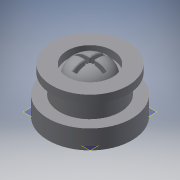
# Autodesk Inventor part: AX12_Idler
Saved by Autodesk Inventor 2017 (Build 210142000, 142)
## iProperties
Created: 2016-09-05
Part Number: AX12_Idler
Material: Generic
Document SubType Name: Modeling
Designer: Labtech
Density: 1 g/cm^3
Appearance: Default
Author: Labtech
Autodesk Inventor part; units mm, degrees
ref_plane "YZ Plane" through (0, 0, 0) normal (1, 0, 0) x (0, 1, 0)
ref_plane "XZ Plane" through (0, 0, 0) normal (0, 1, 0) x (-1, 0, 0)
sketch "Sketch1" plane through (0, 0, 0) normal (0, 0, 1) x (1, 0, 0)
  circle A0 centre (0, 0) radius 4 projected
  circle A1 centre (0, 0) radius 1.625 projected
  point P0 (0, 0)
ref_plane "Work Plane1" through (-11.5847, -11.5847, 5.5) normal (0, 0, 1) x (0.9999727, 0.0073902, 0)
extrude "Extrusion1" add sketch "Sketch1" along normal up to surface (5.5 mm away)
sketch "Sketch2" plane through (0, 0, 5.5) normal (0, 0, 1) x (1, 0, 0)
  circle A0 centre (0, 0) radius 3
  circle A1 centre (0, 0) radius 5
  dimension "d2" = 6
  dimension "d3" = 10
  constraints: 2 centre point, 2 coincident
  measures "d2" diameter of A0
  measures "d3" diameter of A1
extrude "Extrusion2" add sketch "Sketch2" along normal blind 1
ref_plane "Work Plane2" through (0, 0, 1) normal (0, 0, -1) x (-1, 0, 0)
sketch "Sketch3" plane through (0, 0, 1) normal (0, 0, -1) x (-1, 0, 0)
  circle A0 centre (0, 0) radius 4 projected
  circle A1 centre (0, 0) radius 4
  circle A2 centre (0, 0) radius 5.5
  point P0 (0, 0)
  dimension "d7" = 11
  constraints: 2 centre point, 2 coincident
  measures "d7" diameter of A2
extrude "Extrusion3" add sketch "Sketch3" along normal blind 0.5 and the other way blind 2
sketch "Sketch4" plane through (0, 0, 5.5) normal (0, 0, 1) x (1, 0, 0)
  circle A0 centre (0, 0) radius 2.7
  dimension "d12" = 5.4
  constraints: 1 centre point, 1 coincident
  measures "d12" diameter of A0
extrude "Extrusion4" add sketch "Sketch4" along normal blind 1.5
fillet "Fillet1" radius 2 1 edges at (-2.7, 0, 7)
sketch "Sketch5" plane through (0, 0, 7) normal (0, 0, 1) x (1, 0, 0)
  line L0 (0.25, 2) -> (-0.25, 2)
  line L1 (-0.25, 2) -> (-0.25, -2)
  line L2 (-0.25, -2) -> (0.25, -2)
  line L3 (0.25, -2) -> (0.25, 2)
  line L4 (0.25, 2) -> (-0.25, -2) construction
  line L5 (-0.25, 2) -> (0.25, -2) construction
  line L6 (2, 0.25) -> (-2, 0.25)
  line L7 (-2, 0.25) -> (-2, -0.25)
  line L8 (-2, -0.25) -> (2, -0.25)
  line L9 (2, -0.25) -> (2, 0.25)
  line L10 (2, 0.25) -> (-2, -0.25) construction
  line L11 (-2, 0.25) -> (2, -0.25) construction
  point P0 (0, 0)
  dimension "d16" = 0.5
  dimension "d17" = 4
  dimension "d18" = 4
  dimension "d19" = 0.5
  constraints: 24 end point, 4 midpoint, 4 parallel, 2 horizontal, 2 perpendicular
  measures "d16" distance of L2.end L1.end
  measures "d17" distance of L1.end L0.end
  measures "d18" distance of L8.end L7.end
  measures "d19" distance of L7.end L6.end
extrude "Extrusion5" cut sketch "Sketch5" against normal blind 1
chamfer "Chamfer1" distance 0.1 angle 45 16 edges at (0.4857, -0.25, 7) (1.3929, -0.25, 6.8909) (0.4857, 0.25, 7) (1.3929, 0.25, 6.8909) (0.25, -1.3929, 6.8909) (0.25, -0.4857, 7) (-0.25, -1.3929, 6.8909) (-0.25, -0.4857, 7) (-1.3929, -0.25, 6.8909) (-0.4857, -0.25, 7) (-1.3929, 0.25, 6.8909) (-0.4857, 0.25, 7) (-0.25, 1.3929, 6.8909) (-0.25, 0.4857, 7) (0.25, 1.3929, 6.8909) (0.25, 0.4857, 7)
chamfer "Chamfer2" distance 0.1 angle 45 5 edges at (-0.25, 0.25, 6.45) (-0.3, 0.3, 6.95) (-0.25, -0.25, 6.45) (0.25, 0.25, 6.45) (0.25, -0.25, 6.45)
chamfer "Chamfer3" distance 0.1 angle 45 3 edges at (-0.325, -0.325, 6.975) (0.325, -0.325, 6.975) (0.325, 0.325, 6.975)
chamfer "Chamfer4" distance 0.1 angle 45 5 edges at (-0.0112, 2, 6.5719) (2, 0.1292, 6.5687) (2, -0.1292, 6.5687) (0.0112, -2, 6.5719) (-2, -0.0112, 6.5719)
body "Solid1"
